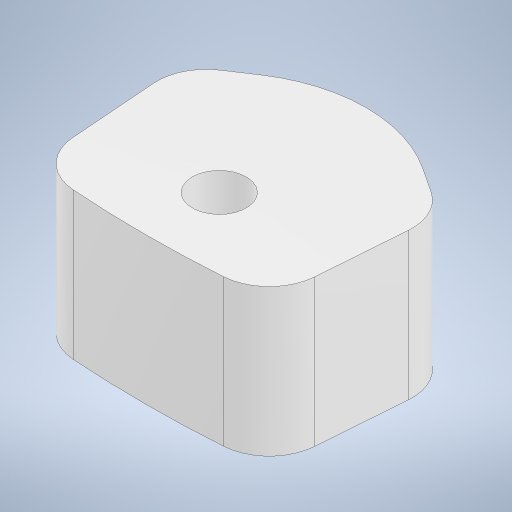
# Autodesk Inventor part: Retaining Ring
Saved by Autodesk Inventor 2023.2 (Build 272271000, 271)
## iProperties
Created: 2022-12-28
Part Number: Retaining Ring
Material: UHMW, White
Document SubType Name: Modeling
Designer: Nathan Cai
Mass: 43.1017 g
Surface Area: 259.691 cm^2
Volume: 45.8529 cm^3
Density: 0.94 g/cm^3
Appearance: Smooth - White
Author: Nathan Cai
Autodesk Inventor part; units mm, degrees
ref_plane "YZ Plane" through (0, 0, 0) normal (1, 0, 0) x (0, 1, 0)
ref_plane "XZ Plane" through (0, 0, 0) normal (0, 1, 0) x (-1, 0, 0)
ref_plane "XY Plane" through (0, 0, 0) normal (0, 0, 1) x (1, 0, 0)
sketch "Sketch1" plane through (0, 0, 0) normal (0, 1, 0) x (-1, 0, 0)
  circle A0 centre (0, 0) radius 73.025
  circle A1 centre (0, 0) radius 84.1375
  line L0 (0, 0) -> (0, 84.1375) construction
  circle A2 centre (0, 65.0875) radius 1.7526
  circle A3 centre (0, 65.0875) radius 7.9375 construction
  circle A4 centre (-61.9019, 20.1131) radius 1.7526
  circle A5 centre (-61.9019, 20.1131) radius 7.9375 construction
  circle A6 centre (-38.2575, -52.6569) radius 1.7526
  circle A7 centre (-38.2575, -52.6569) radius 7.9375 construction
  circle A8 centre (38.2575, -52.6569) radius 1.7526
  circle A9 centre (38.2575, -52.6569) radius 7.9375 construction
  circle A10 centre (61.9019, 20.1131) radius 1.7526
  circle A11 centre (61.9019, 20.1131) radius 7.9375 construction
  arc A12 (-29.3651, -56.0703) -> (-44.2517, -45.2546) centre (-38.2575, -52.6569) ccw
  line L1 (-29.3651, -56.0703) -> (-32.8726, -65.2077)
  line L2 (-44.2517, -45.2546) -> (-51.858, -51.414)
  arc A13 (44.2517, -45.2546) -> (29.3651, -56.0703) centre (38.2575, -52.6569) ccw
  line L3 (29.3651, -56.0703) -> (32.8726, -65.2077)
  line L4 (44.2517, -45.2546) -> (51.858, -51.414)
  arc A14 (-5.2592, 57.1461) -> (5.2592, 57.1461) centre (0, 65.0875) ccw
  arc A15 (55.1667, 26.8483) -> (61.9019, 10.5881) centre (61.9019, 20.1131) ccw
  line L5 (61.9019, 10.5881) -> (72.2533, 10.5881)
  line L6 (0, 0) -> (61.9019, 20.1131) construction
  line L7 (55.1667, 26.8483) -> (63.8164, 35.4981)
  arc A16 (-61.9019, 10.5881) -> (-55.1667, 26.8483) centre (-61.9019, 20.1131) ccw
  line L8 (-61.9019, 10.5881) -> (-72.2533, 10.5881)
  line L9 (-55.1667, 26.8483) -> (-63.8164, 35.4981)
  line L10 (0, 0) -> (12.6807, 71.9156) construction
  circle A17 centre (11.8537, 67.2254) radius 3.3655
  circle A18 centre (0, 0) radius 68.2625 construction
  circle A19 centre (11.8537, 67.2254) radius 4.7625 construction
  circle A20 centre (-11.8537, 67.2254) radius 3.3655
  circle A21 centre (-11.8537, 67.2254) radius 4.7625 construction
  line L11 (-5.2592, 57.1461) -> (-23.4145, 69.1694)
  line L12 (5.2592, 57.1461) -> (23.4145, 69.1694)
  line L13 (7.9375, -79.375) -> (-7.9375, -79.375)
  line L14 (-7.9375, -79.375) -> (-7.9375, -73.025)
  line L15 (-7.9375, -73.025) -> (7.9375, -73.025)
  line L16 (7.9375, -73.025) -> (7.9375, -79.375)
  line L17 (7.9375, -79.375) -> (-7.9375, -73.025) construction
  line L18 (-7.9375, -79.375) -> (7.9375, -73.025) construction
  line L19 (0, -76.2) -> (0, -84.1375) construction
  line L20 (12.7, -82.55) -> (-12.7, -82.55) construction
  line L21 (-12.7, -82.55) -> (-12.7, -69.85)
  line L22 (-12.7, -69.85) -> (12.7, -69.85)
  line L23 (12.7, -69.85) -> (12.7, -82.55)
  line L24 (12.7, -82.55) -> (-12.7, -69.85) construction
  line L25 (-12.7, -82.55) -> (12.7, -69.85) construction
  line L26 (30.7823, -63.9747) -> (51.3313, -49.045)
  line L27 (36.5014, -63.744) -> (49.3446, -54.4129)
  line L28 (53.077, -59.5502) -> (40.2339, -68.8813)
  line L29 (40.2339, -68.8813) -> (36.5014, -63.744)
  line L30 (49.3446, -54.4129) -> (53.077, -59.5502)
  line L31 (53.077, -59.5502) -> (36.5014, -63.744) construction
  line L32 (40.2339, -68.8813) -> (49.3446, -54.4129) construction
  line L33 (51.3313, -49.045) -> (58.7962, -59.3195)
  line L34 (58.7962, -59.3195) -> (38.2472, -74.2492) construction
  line L35 (38.2472, -74.2492) -> (51.3313, -49.045) construction
  line L36 (58.7962, -59.3195) -> (30.7823, -63.9747) construction
  line L37 (38.2472, -74.2492) -> (30.7823, -63.9747)
  line L38 (62.5068, -33.6633) -> (70.3558, -9.5064)
  line L39 (66.9981, -30.115) -> (71.9037, -15.017)
  line L40 (77.9429, -16.9792) -> (73.0373, -32.0772)
  line L41 (73.0373, -32.0772) -> (66.9981, -30.115)
  line L42 (71.9037, -15.017) -> (77.9429, -16.9792)
  line L43 (77.9429, -16.9792) -> (66.9981, -30.115) construction
  line L44 (73.0373, -32.0772) -> (71.9037, -15.017) construction
  line L45 (70.3558, -9.5064) -> (82.4342, -13.4309)
  line L46 (82.4342, -13.4309) -> (74.5852, -37.5878) construction
  line L47 (74.5852, -37.5878) -> (70.3558, -9.5064) construction
  line L48 (82.4342, -13.4309) -> (62.5068, -33.6633) construction
  line L49 (74.5852, -37.5878) -> (62.5068, -33.6633)
  line L50 (70.3558, 9.5064) -> (62.5068, 33.6633)
  line L51 (71.9037, 15.017) -> (66.9981, 30.115)
  line L52 (73.0373, 32.0772) -> (77.9429, 16.9792)
  line L53 (77.9429, 16.9792) -> (71.9037, 15.017)
  line L54 (66.9981, 30.115) -> (73.0373, 32.0772)
  line L55 (73.0373, 32.0772) -> (71.9037, 15.017) construction
  line L56 (77.9429, 16.9792) -> (66.9981, 30.115) construction
  line L57 (62.5068, 33.6633) -> (74.5852, 37.5878)
  line L58 (74.5852, 37.5878) -> (82.4342, 13.4309) construction
  line L59 (82.4342, 13.4309) -> (62.5068, 33.6633) construction
  line L60 (74.5852, 37.5878) -> (70.3558, 9.5064) construction
  line L61 (82.4342, 13.4309) -> (70.3558, 9.5064)
  line L62 (51.3313, 49.045) -> (30.7823, 63.9747)
  line L63 (49.3446, 54.4129) -> (36.5014, 63.744)
  line L64 (40.2339, 68.8813) -> (53.077, 59.5502)
  line L65 (53.077, 59.5502) -> (49.3446, 54.4129)
  line L66 (36.5014, 63.744) -> (40.2339, 68.8813)
  line L67 (40.2339, 68.8813) -> (49.3446, 54.4129) construction
  line L68 (53.077, 59.5502) -> (36.5014, 63.744) construction
  line L69 (30.7823, 63.9747) -> (38.2472, 74.2492)
  line L70 (38.2472, 74.2492) -> (58.7962, 59.3195) construction
  line L71 (58.7962, 59.3195) -> (30.7823, 63.9747) construction
  line L72 (38.2472, 74.2492) -> (51.3313, 49.045) construction
  line L73 (58.7962, 59.3195) -> (51.3313, 49.045)
  circle A22 centre (0, 0) radius 69.85
  line L74 (17.6671, 70.8557) -> (16.0268, 64.2769)
  line L75 (-17.6671, 70.8557) -> (-16.0268, 64.2769)
  line L76 (-38.2575, -52.6569) -> (-49.4548, -68.0687) construction
  line L77 (12.7, 69.85) -> (-12.7, 69.85)
  line L78 (7.9375, 73.025) -> (-7.9375, 73.025)
  line L79 (-7.9375, 79.375) -> (7.9375, 79.375)
  line L80 (7.9375, 79.375) -> (7.9375, 73.025)
  line L81 (-7.9375, 73.025) -> (-7.9375, 79.375)
  line L82 (-7.9375, 79.375) -> (7.9375, 73.025) construction
  line L83 (7.9375, 79.375) -> (-7.9375, 73.025) construction
  line L84 (-12.7, 69.85) -> (-12.7, 82.55)
  line L85 (-12.7, 82.55) -> (12.7, 82.55) construction
  line L86 (12.7, 82.55) -> (-12.7, 69.85) construction
  line L87 (-12.7, 82.55) -> (12.7, 69.85) construction
  line L88 (12.7, 82.55) -> (12.7, 69.85)
  line L89 (-30.7823, 63.9747) -> (-51.3313, 49.045)
  line L90 (-36.5014, 63.744) -> (-49.3446, 54.4129)
  line L91 (-53.077, 59.5502) -> (-40.2339, 68.8813)
  line L92 (-40.2339, 68.8813) -> (-36.5014, 63.744)
  line L93 (-49.3446, 54.4129) -> (-53.077, 59.5502)
  line L94 (-53.077, 59.5502) -> (-36.5014, 63.744) construction
  line L95 (-40.2339, 68.8813) -> (-49.3446, 54.4129) construction
  line L96 (-51.3313, 49.045) -> (-58.7962, 59.3195)
  line L97 (-58.7962, 59.3195) -> (-38.2472, 74.2492) construction
  line L98 (-38.2472, 74.2492) -> (-51.3313, 49.045) construction
  line L99 (-58.7962, 59.3195) -> (-30.7823, 63.9747) construction
  line L100 (-38.2472, 74.2492) -> (-30.7823, 63.9747)
  line L101 (-62.5068, 33.6633) -> (-70.3558, 9.5064)
  line L102 (-66.9981, 30.115) -> (-71.9037, 15.017)
  line L103 (-77.9429, 16.9792) -> (-73.0373, 32.0772)
  line L104 (-73.0373, 32.0772) -> (-66.9981, 30.115)
  line L105 (-71.9037, 15.017) -> (-77.9429, 16.9792)
  line L106 (-77.9429, 16.9792) -> (-66.9981, 30.115) construction
  line L107 (-73.0373, 32.0772) -> (-71.9037, 15.017) construction
  line L108 (-70.3558, 9.5064) -> (-82.4342, 13.4309)
  line L109 (-82.4342, 13.4309) -> (-74.5852, 37.5878) construction
  line L110 (-74.5852, 37.5878) -> (-70.3558, 9.5064) construction
  line L111 (-82.4342, 13.4309) -> (-62.5068, 33.6633) construction
  line L112 (-74.5852, 37.5878) -> (-62.5068, 33.6633)
  line L113 (-70.3558, -9.5064) -> (-62.5068, -33.6633)
  line L114 (-71.9037, -15.017) -> (-66.9981, -30.115)
  line L115 (-73.0373, -32.0772) -> (-77.9429, -16.9792)
  line L116 (-77.9429, -16.9792) -> (-71.9037, -15.017)
  line L117 (-66.9981, -30.115) -> (-73.0373, -32.0772)
  line L118 (-73.0373, -32.0772) -> (-71.9037, -15.017) construction
  line L119 (-77.9429, -16.9792) -> (-66.9981, -30.115) construction
  line L120 (-62.5068, -33.6633) -> (-74.5852, -37.5878)
  line L121 (-74.5852, -37.5878) -> (-82.4342, -13.4309) construction
  line L122 (-82.4342, -13.4309) -> (-62.5068, -33.6633) construction
  line L123 (-74.5852, -37.5878) -> (-70.3558, -9.5064) construction
  line L124 (-82.4342, -13.4309) -> (-70.3558, -9.5064)
  line L125 (-51.3313, -49.045) -> (-30.7823, -63.9747)
  line L126 (-49.3446, -54.4129) -> (-36.5014, -63.744)
  line L127 (-40.2339, -68.8813) -> (-53.077, -59.5502)
  line L128 (-53.077, -59.5502) -> (-49.3446, -54.4129)
  line L129 (-36.5014, -63.744) -> (-40.2339, -68.8813)
  line L130 (-40.2339, -68.8813) -> (-49.3446, -54.4129) construction
  line L131 (-53.077, -59.5502) -> (-36.5014, -63.744) construction
  line L132 (-30.7823, -63.9747) -> (-38.2472, -74.2492)
  line L133 (-38.2472, -74.2492) -> (-58.7962, -59.3195) construction
  line L134 (-58.7962, -59.3195) -> (-30.7823, -63.9747) construction
  line L135 (-38.2472, -74.2492) -> (-51.3313, -49.045) construction
  line L136 (-58.7962, -59.3195) -> (-51.3313, -49.045)
  line L137 (7.633, 69.4317) -> (8.401, 59.2267)
  line L138 (-7.633, 69.4317) -> (-8.401, 59.2267)
  point P0 (51.858, -51.414)
  point P1 (64.5887, 34.0727)
  point P2 (44.7892, -61.6471)
  point P3 (72.4705, -23.5471)
  point P4 (72.4705, 23.5471)
  point P5 (44.7892, 61.6471)
  point P6 (12.7, -71.9122)
  point P7 (-12.7, -71.9122)
  point P8 (31.9944, 65.643)
  point P9 (52.5434, 50.7133)
  point P10 (64.468, 34.3005)
  point P11 (72.3171, 10.1437)
  point P12 (72.3171, -10.1437)
  point P13 (64.468, -34.3005)
  point P14 (52.5434, -50.7133)
  point P15 (31.9944, -65.643)
  point P16 (66.4313, 21.5848)
  point P17 (-20.018, 66.9201)
  point P18 (-61.4776, 33.1592)
  point P19 (20.018, 66.9201)
  point P20 (66.4313, -21.5848)
  point P21 (61.4776, 33.1592)
  point P22 (41.0568, -56.5098)
  point P23 (69.0428, 10.5881)
  point P24 (49.3775, -49.4053)
  point P25 (41.0568, 56.5098)
  point P26 (-69.0428, 10.5881)
  point P27 (-49.3775, -49.4053)
  point P28 (31.7288, -62.2279)
  point P29 (0, -69.85)
  point P30 (-31.7288, -62.2279)
  point P31 (0, 76.2)
  point P32 (-44.7892, 61.6471)
  point P33 (-72.4705, 23.5471)
  point P34 (-72.4705, -23.5471)
  point P35 (-44.7892, -61.6471)
  point P36 (32.0467, -63.0561)
  point P37 (50.0669, -49.9636)
  point P38 (70.0043, 10.5881)
  point P39 (62.7968, 32.7708)
  point P40 (12.7, 71.9122)
  point P41 (12.7, 70.4828)
  point P42 (9.1625, 69.2464)
  point P43 (-9.1625, 69.2464)
  point P44 (-12.7, 70.4828)
  point P45 (-12.7, 71.9122)
  point P46 (16.899, 67.775)
  point P47 (15.0737, 68.2041)
  point P48 (-15.0737, 68.2041)
  point P49 (-16.899, 67.775)
  dimension "d1" = 146.05
  dimension "d13" = 136.525
  dimension "d14" = 9.525
  dimension "d78" = 3.175
  dimension "d0" = 11.1125
  dimension "d2" = 3.5052
  dimension "d3" = 15.875
  dimension "d6" = 360
  dimension "d8" = 19.05
  dimension "d9" = 19.05
  dimension "d10" = 19.05
  dimension "d11" = 10
  dimension "d12" = 6.731
  dimension "d34" = 15.875
  dimension "d35" = 6.35
  dimension "d37" = 25.4
  dimension "d39" = 3.175
  dimension "d42" = 360
  dimension "d151" = 76.2
  dimension "d153" = 15
  dimension "d163" = 90
  constraints: 278 end point, 19 centre point, 18 symmetric about line, 13 coincident, 13 point on circle, 7 point on line, 7 tangent, 4 midpoint, 4 parallel, 3 perpendicular, 2 horizontal, 2 vertical, 258 other
  measures "d2" diameter of A2
  measures "d3" diameter of A3
  measures "d8" diameter of A12
  measures "d9" diameter of A14
  measures "d10" diameter of A15
  measures "d11" angle of L0 L10
  measures "d12" diameter of A17
  measures "d34" distance of L14.end L15.end
  measures "d35" distance of L13.end L14.end
  measures "d37" distance of L21.end L22.end
  measures "d39" distance between parallel lines of L15 L22
  measures "d151" distance of point (0, 0) L19.start
  measures "d153" angle of L76 L1
  measures "d163" angle of L9 L7
extrude "Extrusion1" add sketch "Sketch1" along normal blind 9.525 contours L12 A14 L11 L138 A22 L137
fillet "Fillet14" radius 3.175 4 edges at (-7.633, 4.7625, 69.4317) (-8.401, 4.7625, 59.2267) (8.401, 4.7625, 59.2267) (7.633, 4.7625, 69.4317)
equation "\"d1\" = Ring_ID"
equation "\"BearingTol\" = 0.1"
equation "\"CSDepth\" = 1.7272"
equation "\"CSAngle\" = 41deg"
equation "\"Ring_ID\" = 146.05"
body "Solid1"
